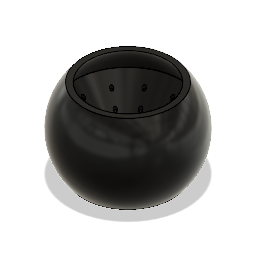
pot (Autodesk Fusion 360 design; units mm, degrees)
Autodesk Fusion 360 part; units mm, degrees
note: some values were not read from the file. Set by a fixed rule: which sketch regions a step uses.
sketch "Sketch1" plane through (0, 0, 0) normal (1, 0, 0) x (0, 0, -1)
  circle A0 centre (0, 0) radius 60
  line L0 (-60, 0) -> (60, 0) construction
  line L1 (-48.734, -35) -> (48.734, -35)
  line L2 (-44.7214, 40) -> (44.7214, 40)
  line L3 (0, 0) -> (0, 40) construction
  line L4 (12, -35) -> (53.954, 14.9988)
  line L5 (0, -35) -> (43.715, -35) construction
  line L6 (22, -26.1939) -> (54.5615, 12.6113)
  line L7 (22, -35) -> (22, -26.1939)
  line L8 (55.0624, 23.8354) -> (54.5836, 23.8354)
  circle A1 centre (0, 0) radius 56
  line L9 (0, 0) -> (0, -35) construction
  line L10 (-44.7214, -40) -> (44.7214, -40)
  line L11 (0, -35) -> (0, -40)
  point P0 (0, 20.572)
  dimension "d1" = 120
  dimension "d2" = 35
  dimension "d3" = 40
  dimension "d4" = 50
  dimension "d5" = 2
  dimension "d7" = 112
  dimension "d8" = 12
  dimension "d9" = 10
  dimension "d10" = 5
  constraint coincident A0.centre L3.start
  constraint coincident A0 L0.start
  constraint coincident A0 L0.end
  constraint horizontal L0
  constraint coincident A0 L1.start
  constraint coincident A0 L1.end
  constraint horizontal L1
  constraint coincident A0 L2.start
  constraint coincident A0 L2.end
  constraint horizontal L2
  constraint midpoint L2 L3.end
  constraint horizontal L5
  constraint coincident A0 L8.start
  constraint coincident L5 L7.start
  constraint perpendicular L5 L7
  constraint coincident L6.start L7
  constraint horizontal L8
  constraint coincident L5.end A1
  constraint coincident A1 L6.end
  constraint coincident L1 L7.start
  constraint parallel L3 L9
  constraint coincident L5 L4.start
  constraint coincident A0 L10.start
  constraint coincident A0 L10.end
  constraint horizontal L10
  constraint midpoint L10 L11.end
  constraint coincident A1 L4.end
  measures "d1" diameter of A0
  measures "d2" distance of A0.centre L5.start
  measures "d3" distance of A0.centre L3.end
  measures "d4" angle of L4 L5
  measures "d5" distance of L4 L6
  measures "d7" diameter of A1
  measures "d8" distance of L5.start L4.start
  measures "d9" distance of L7.start L4.start
  measures "d10" distance of L1 L10
revolve "Revolve1" add sketch "Sketch1" angle 360 about axis through (0, 0, 0) along (0, 1, 0) contours A0 L1 L2 A1 | A0 L1 A1 L10 | L1 A1 L10 L11 | L1 L4 L6 L7 A1 picked at (46.8259, -32.9322) picked at (44.0359, -36.7027) picked at (20.3973, -38.3333)
ref_plane "WorkPlane1" through (0, 20.572, 0) normal (0, 1, 0) x (1, 0, 0)
sketch "Sketch5" plane through (0, 20.572, 0) normal (0, 1, 0) x (1, 0, 0)
  circle A0 centre (0, 0) radius 55
  line L0 (0, 0) -> (0, 25) construction
  line L1 (0, 0) -> (0, 1.4124) construction
  line L2 (0, 35) -> (0, 0) construction
  line L3 (0, 45) -> (0, 0) construction
  circle A1 centre (0, 25) radius 1.5
  circle A2 centre (0, 35) radius 1.5
  circle A3 centre (0, 45) radius 1.5
  circle A4 centre (0, 0) radius 12
  circle A5 centre (0, 0) radius 17
  point P0 (0, 12)
  dimension "d15" = 110
  dimension "d16" = 25
  dimension "d17" = 35
  dimension "d18" = 45
  dimension "d19" = 3
  dimension "d20" = 3
  dimension "d21" = 3
  dimension "d30" = 34
  constraint coincident A0.centre L0.start
  constraint vertical L0
  constraint coincident L0 L1.end
  constraint parallel L1 L2
  constraint parallel L0 L3
  constraint coincident L0.end A1.centre
  constraint coincident L2.start A2.centre
  constraint coincident L3.start A3.centre
  constraint concentric A0 A4
  constraint coincident A4 P0
  constraint concentric A0 A5
  measures "d15" diameter of A0
  measures "d16" distance of A0.centre L0.end
  measures "d17" distance of A0.centre L2.start
  measures "d18" distance of L3.start A0.centre
  measures "d19" diameter of A1
  measures "d20" diameter of A2
  measures "d21" diameter of A3
  measures "d30" diameter of A5
extrude "Extrude1" cut sketch "Sketch5" against normal blind 50 contours A1
extrude "Extrude2" cut sketch "Sketch5" against normal blind 45 contours A2
extrude "Extrude3" cut sketch "Sketch5" against normal blind 40 contours A3
pattern_circular "C-Pattern1" count 12 over 360 about axis through (0, 1.75, 0) along (0, 1, 0) of "Extrude1", "Extrude2", "Extrude3"
equation "d30 = 24 mm + 10 mm"
